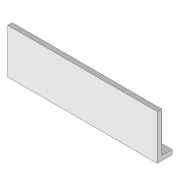
# Autodesk Inventor part: Seitboard
Saved by Autodesk Inventor 2020 (Build 240168000, 168)
## iProperties
Created: 2020-03-18
Part Number: Seitboard
Material: Generisch
Document SubType Name: Modeling
Designer: franz
Density: 1 g/cm^3
Appearance: Vorgabe
Author: franz
Autodesk Inventor part; units mm, degrees
ref_plane "YZ Plane" through (0, 0, 0) normal (1, 0, 0) x (0, 1, 0)
ref_plane "XZ Plane" through (0, 0, 0) normal (0, 1, 0) x (-1, 0, 0)
ref_plane "XY Plane" through (0, 0, 0) normal (0, 0, 1) x (1, 0, 0)
sketch "Skizze1" plane through (0, 0, 0) normal (1, 0, 0) x (0, 1, 0)
  line L0 (0, 0) -> (0, -100)
  line L1 (0, -100) -> (30, -100)
  line L2 (30, -100) -> (30, -30)
  line L3 (30, -30) -> (300, -30)
  line L4 (300, -30) -> (300, 0)
  line L5 (300, 0) -> (0, 0)
  dimension "d0" = 100
  dimension "d1" = 300
  dimension "d2" = 30
  dimension "d3" = 30
  constraints: 12 end point, 5 perpendicular, 1 vertical
  measures "d0" distance of L0.start L0.end
  measures "d1" distance of L4.end L0.start
  measures "d2" distance of L0.end L1.end
  measures "d3" distance of L3.end L4.end
extrude "Extrusion1" add sketch "Skizze1" along normal blind 1300
equation "\"d3\" = d2"
